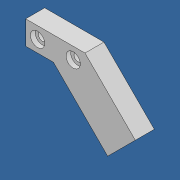
# Autodesk Inventor part: Sensor_Holder
Saved by Autodesk Inventor 2020 (Build 240168000, 168)
## iProperties
Created: 2021-05-07
Part Number: Sensor_Holder
Material: 一般
Document SubType Name: Modeling
Designer: ken113
Density: 1 g/cm^3
Appearance: 既定
Author: ken113
Autodesk Inventor part; units mm, degrees
ref_plane "YZ Plane" through (0, 0, 0) normal (1, 0, 0) x (0, 1, 0)
ref_plane "XZ Plane" through (0, 0, 0) normal (0, 1, 0) x (-1, 0, 0)
ref_plane "XY Plane" through (0, 0, 0) normal (0, 0, 1) x (1, 0, 0)
sketch "スケッチ1" plane through (0, 0, 0) normal (0, 0, 1) x (1, 0, 0)
  line L0 (-15, 0) -> (10, 0)
  line L1 (10, 0) -> (10, 10)
  line L2 (10, 10) -> (-15, 10)
  line L3 (-15, 10) -> (-15, 0)
  point P0 (0, 0)
  dimension "d0" = 10
  dimension "d1" = 25
  dimension "d2" = 15
  constraints: 8 end point, 2 parallel, 1 horizontal, 1 perpendicular
  measures "d0" distance of L0.end L1.end
  measures "d1" distance of L1.end L2.end
  measures "d2" distance from line of point (0, 0) L3
extrude "押し出し1" add sketch "スケッチ1" along normal blind 8
sketch "スケッチ2" plane through (0, 0, 8) normal (0, 0, 1) x (1, 0, 0)
  line L0 (10, 0) -> (10, 10) projected
  line L1 (10, 10) -> (-15, 10) projected
  line L2 (-15, 10) -> (-15, 0) projected
  line L3 (-15, 0) -> (10, 0) projected
  point P0 (0, 0)
  point P1 (-10, 5)
  point P2 (5, 5)
  dimension "d6" = 5
  dimension "d7" = 5
  dimension "d15" = 5
  constraints: 1 horizontal alignment
  measures "d6" distance from line of L0 point (5, 5)
  measures "d7" distance from line of point (-10, 5) L1
  measures "d15" distance from line of point (-10, 5) L2
hole "穴1" at (-10, 5, 8) at (5, 5, 8) direction (0, 0, -1) diameter 3.3 end through all counterbore diameter 6 counterbore depth 2
sketch "スケッチ3" plane through (0, 0, 8) normal (0, 0, 1) x (1, 0, 0)
  circle A0 centre (-10, 5) radius 3 projected
  circle A1 centre (5, 5) radius 3 projected
  line L0 (10, 10) -> (-15, 10) projected
  line L1 (-15, 10) -> (-15, 0) projected
  line L2 (-15, 0) -> (10, 0) projected
  line L3 (10, 0) -> (10, 10) projected
  line L4 (10, 10) -> (-15, 10) projected
  line L5 (10, 10) -> (31.2132, -11.2132)
  line L6 (31.2132, -11.2132) -> (19.5572, -22.8692)
  line L7 (19.5572, -22.8692) -> (-3.312, 0)
  point P0 (0, 0)
  dimension "d16" = 45
  dimension "d17" = 30
  constraints: 6 end point, 1 parallel, 1 perpendicular, 1 point on line
  measures "d16" angle of L5 L3
  measures "d17" distance from line of L6 A1.centre
extrude "押し出し2" add sketch "スケッチ3" against normal blind 8 contours L5 L6 L7 L2 L3
